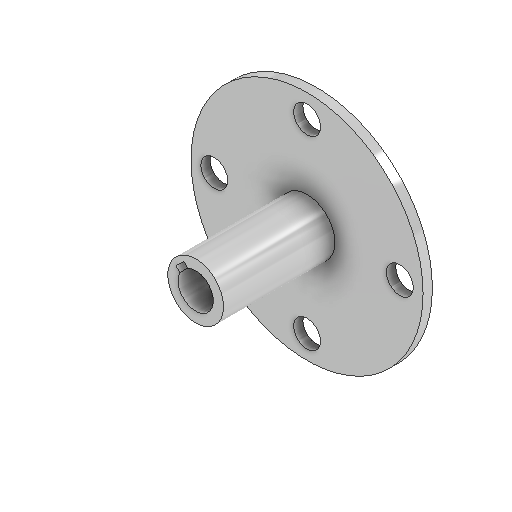
# Autodesk Inventor part: wheelFlangeMotor
Saved by Autodesk Inventor 2022 (Build 260153000, 153)
## iProperties
Created: 2024-07-01
Part Number: wheelFlangeMotor
Material: Generic
Document SubType Name: Modeling
Designer: LaptopJR
Density: 1 g/cm^3
Appearance: Aluminum - Dark
Author: LaptopJR
Autodesk Inventor part; units mm, degrees
ref_plane "YZ Plane" through (0, 0, 0) normal (1, 0, 0) x (0, 1, 0)
ref_plane "XZ Plane" through (0, 0, 0) normal (0, 1, 0) x (-1, 0, 0)
ref_plane "XY Plane" through (0, 0, 0) normal (0, 0, 1) x (1, 0, 0)
sketch "Sketch1" plane through (0, 0, 0) normal (0, 0, 1) x (1, 0, 0)
  circle A0 centre (0, 0) radius 50 construction
  circle A1 centre (0, 50) radius 7.25
  circle A2 centre (-50, 0) radius 7.25
  circle A3 centre (0, -50) radius 7.25
  circle A4 centre (50, 0) radius 7.25
  circle A5 centre (0, 0) radius 15 construction
  circle A6 centre (0, 0) radius 62.5
  circle A7 centre (0, 0) radius 9.5
  dimension "d0" = 100
  dimension "d1" = 14.5
  dimension "d4" = 360
  dimension "d6" = 30
  dimension "d7" = 125
  dimension "d8" = 19
  constraints: 7 centre point, 4 coincident, 1 vertical alignment, 11 other
  measures "d1" diameter of A1
  measures "d6" diameter of A5
  measures "d7" diameter of A6
  measures "d8" diameter of A7
extrude "Extrusion1" add sketch "Sketch1" along normal blind 5
sketch "Sketch2" plane through (0, 0, 5) normal (0, 0, 1) x (1, 0, 0)
  circle A0 centre (0, 0) radius 15
  circle A1 centre (0, 0) radius 9.5 projected
  dimension "d11" = 30
  constraints: 1 centre point, 1 coincident
  measures "d11" diameter of A0
extrude "Extrusion2" add sketch "Sketch2" along normal blind 60
sketch "Sketch3" plane through (0, 0, 65) normal (0, 0, 1) x (1, 0, 0)
  circle A0 centre (0, 0) radius 15 projected
  circle A1 centre (0, 0) radius 9.5 projected
  line L0 (6.7175, -6.7175) -> (-8.4853, 8.4853)
  line L1 (-8.4853, 8.4853) -> (-10.6066, 6.364)
  line L2 (-10.6066, 6.364) -> (-8.4951, 4.2525)
  line L3 (-8.4853, 8.4853) -> (-6.364, 10.6066)
  line L4 (-6.364, 10.6066) -> (-4.2525, 8.4951)
  dimension "d14" = 21.5
  dimension "d15" = 3
  dimension "d16" = 3
  constraints: 10 end point, 2 perpendicular
  measures "d14" distance of L0.start L0.end
  measures "d15" distance of L0.end L1.end
  measures "d16" distance of L0.end L3.end
extrude "Extrusion3" cut sketch "Sketch3" against normal blind 40 contours A1 L0 L3 L4 | A1 L2 L1 L0
body "Solid1"
